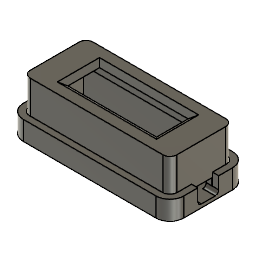
Slot na displej (Autodesk Fusion 360 design; units mm, degrees)
Autodesk Fusion 360 part; units mm, degrees
sketch "Sketch1" plane through (0, 0, 0) normal (0, 0, 1) x (1, 0, 0)
  line L0 (19.5, 10.25) -> (-18.5, 10.25)
  line L1 (-20.5, 8.25) -> (-20.5, -5.75)
  line L2 (-18.5, -7.75) -> (19.5, -7.75)
  line L3 (21.5, -5.75) -> (21.5, 8.25)
  line L4 (21.5, 10.25) -> (-20.5, -7.75) construction
  line L5 (-20.5, 10.25) -> (21.5, -7.75) construction
  line L6 (19.2, 6.275) -> (-19.2, 6.275)
  line L7 (-19.2, 6.275) -> (-19.2, -6.275)
  line L8 (-19.2, -6.275) -> (19.2, -6.275)
  line L9 (19.2, 6.275) -> (-19.2, -6.275) construction
  line L10 (-19.2, 6.275) -> (19.2, -6.275) construction
  arc A0 (21.5, 8.25) -> (19.5, 10.25) centre (19.5, 8.25) ccw
  arc A1 (19.5, -7.75) -> (21.5, -5.75) centre (19.5, -5.75) ccw
  arc A2 (-20.5, -5.75) -> (-18.5, -7.75) centre (-18.5, -5.75) ccw
  arc A3 (-18.5, 10.25) -> (-20.5, 8.25) centre (-18.5, 8.25) ccw
  line L11 (19.2, 2.9246) -> (13.2, 2.9246) construction
  line L12 (-19.2, 0) -> (-12.2, 0) construction
  line L13 (6.4271, 6.275) -> (6.4271, 5.775) construction
  line L14 (3.4944, -6.275) -> (3.4944, -3.275) construction
  line L15 (-12.2, -3.275) -> (13.2, -3.275)
  line L16 (13.2, -3.275) -> (13.2, 5.775)
  line L17 (13.2, 5.775) -> (-12.2, 5.775)
  line L18 (-12.2, 5.775) -> (-12.2, -3.275)
  line L19 (-13.7, -4.775) -> (14.7, -4.775)
  line L20 (14.7, -4.775) -> (14.7, 7.275)
  line L21 (14.7, 7.275) -> (-13.7, 7.275)
  line L22 (-13.7, 7.275) -> (-13.7, -4.775)
  line L23 (19.2, -6.275) -> (19.2, 2.725) construction
  line L24 (19.2, -6.275) -> (19.9, -6.275)
  line L25 (19.9, -6.275) -> (19.9, 2.725)
  line L26 (19.9, 2.725) -> (19.2, 2.725)
  line L27 (19.2, 6.275) -> (19.2, 2.725)
  line L28 (19.2, 6.275) -> (19.2, -6.275) construction
  line L29 (-12.2, -3.275) -> (13.2, 5.775) construction
  line L30 (-12.2, 5.775) -> (13.2, -3.275) construction
  point P0 (0.5, 1.25)
  point P1 (0.5, 1.25)
  dimension "d1" = 42
  dimension "d2" = 18
  dimension "d3" = 38.4
  dimension "d4" = 12.55
  dimension "d5" = 2
  dimension "d6" = 6
  dimension "d7" = 7
  dimension "d8" = 0.5
  dimension "d9" = 3
  dimension "d10" = 1.5
  dimension "d15" = 9
  dimension "d16" = 0.7
  constraint horizontal L0
  constraint perpendicular L0 L1
  constraint parallel L0 L2
  constraint parallel L1 L3
  constraint horizontal L6
  constraint perpendicular L6 L7
  constraint parallel L6 L8
  constraint coincident L9 origin
  constraint coincident L10 origin
  constraint coincident L4.start L0
  constraint coincident L4.start L3
  constraint tangent L0 A0
  constraint tangent L3 A0
  constraint coincident L5.end L3
  constraint coincident L5.end L2
  constraint tangent L3 A1
  constraint tangent L2 A1
  constraint equal A0 A1
  constraint coincident L4.end L2
  constraint coincident L4.end L1
  constraint tangent L2 A2
  constraint tangent L1 A2
  constraint equal A0 A2
  constraint coincident L5.start L1
  constraint coincident L5.start L0
  constraint tangent L1 A3
  constraint tangent L0 A3
  constraint equal A0 A3
  constraint midpoint L7 L12.start
  constraint perpendicular L7 L12
  constraint coincident L6 L13.start
  constraint perpendicular L6 L13
  constraint coincident L8 L14.start
  constraint perpendicular L8 L14
  constraint horizontal L15
  constraint vertical L16
  constraint horizontal L17
  constraint vertical L18
  constraint coincident L13.end L17
  constraint coincident L11.end L16
  constraint coincident L14.end L15
  constraint coincident L12.end L18
  constraint perpendicular L8 L23
  constraint perpendicular L24 L25
  constraint perpendicular L26 L27
  constraint perpendicular L8 L28
  constraint coincident L11.start L28
  constraint perpendicular L11 L16
  constraint perpendicular L25 L26
  constraint midpoint L29 P1
  constraint midpoint L4 P1
  constraint coincident P1 P0
  measures "d1" distance of L4.end L5.end
  measures "d2" distance of L5.start L4.end
  measures "d3" distance of L7.end L8.end
  measures "d4" distance of L6.end L7.end
  measures "d5" radius of A0
  measures "d6" distance of L11.start L11.end
  measures "d7" distance of L12.start L12.end
  measures "d8" distance of L13.start L13.end
  measures "d9" distance of L14.start L14.end
  measures "d15" distance of L8.end L23.end
  measures "d16" distance of L8.end L24.end
extrude "Extrude1" add sketch "Sketch1" against normal blind 1 contours L0 L1 L2 L3 A0 A1 A2 A3 | L6 L7 L8 L19 L20 L22 L24 L25 L26 L27 | L6 L19 L20 L22 | L6 L20 L21 L22 makes body 1
chamfer "Chamfer1" distance 1.5 distance2 1 4 edges at (-12.2, 1.25, 0) (0.5, 5.775, 0) (0.5, -3.275, 0) (13.2, 1.25, 0) measured on face at (-17.7333, 2.7583, 0) measured on face at (-17.7333, 2.7583, 0) measured on face at (-17.7333, 2.7583, 0) measured on face at (-17.7333, 2.7583, 0) on bodies 1
extrude "Extrude2" add sketch "Sketch1" along normal blind -3.2 and the other way blind 1 contours L0 L1 L2 L3 A0 A1 A2 A3 | L6 L20 L21 L22 bodies 1
sketch "Sketch2" plane through (0, 0, -3.2) normal (0, 0, -1) x (1, 0, 0)
  line L0 (-19.2, -6.275) -> (-19.2, 6.275)
  line L1 (-19.2, 6.275) -> (19.9, 6.275)
  line L2 (19.9, 6.275) -> (19.9, -2.725)
  line L3 (19.9, -2.725) -> (19.2, -2.725)
  line L4 (19.2, -2.725) -> (19.2, -6.275)
  line L5 (19.2, -6.275) -> (-19.2, -6.275)
  arc A0 (-20.5, -8.25) -> (-18.5, -10.25) centre (-18.5, -8.25) ccw
  line L6 (-18.5, -10.25) -> (19.5, -10.25)
  arc A1 (19.5, -10.25) -> (21.5, -8.25) centre (19.5, -8.25) ccw
  line L7 (21.5, -8.25) -> (21.5, 5.75)
  arc A2 (21.5, 5.75) -> (19.5, 7.75) centre (19.5, 5.75) ccw
  line L8 (19.5, 7.75) -> (-18.5, 7.75)
  arc A3 (-18.5, 7.75) -> (-20.5, 5.75) centre (-18.5, 5.75) ccw
  line L9 (-20.5, 5.75) -> (-20.5, -8.25)
  line L10 (-19.2, 6.275) -> (-19.2, -8.25)
  line L11 (-19.2, -8.25) -> (19.9, -8.25)
  line L12 (19.9, -8.25) -> (19.9, 6.275)
  line L13 (19.9, 6.275) -> (-19.2, 6.275)
  dimension "d22" = 1.6
  dimension "d23" = 1.3
  dimension "d24" = 2
  measures "d22" distance of L7 L12
  measures "d23" distance of L9 L10
  measures "d24" distance of L6 L11
extrude "Extrude3" add sketch "Sketch2" along normal blind 9.5 bodies 1
chamfer "Chamfer2" distance 2 distance2 2 1 edges at (0.35, 8.25, -3.2) measured on face at (6.6333, 7.5917, -3.2) on bodies 1
chamfer "Chamfer3" distance 0.7 distance2 2 1 edges at (19.9, 4.4875, -3.2) measured on face at (19.4333, 3.9, -3.2) on bodies 1
extrude "Extrude1'" add 1 faces at (-5.9333, 8.9167, -12.7) along direction (0, 0, -1) blind 2 separate body on bodies 1 makes body 2 in component "Component"
sketch "Sketch4" plane through (0, 0, -14.7) normal (0, 0, -1) x (1, 0, 0)
  line L0 (-19.2, 6.275) -> (19.9, 6.275)
  line L1 (19.9, 6.275) -> (19.9, -8.25)
  line L2 (19.9, -8.25) -> (-19.2, -8.25)
  line L3 (-19.2, -8.25) -> (-19.2, 6.275)
  line L4 (-20.5, 5.75) -> (-20.5, -8.25)
  arc A0 (-20.5, -8.25) -> (-18.5, -10.25) centre (-18.5, -8.25) ccw
  line L5 (-18.5, -10.25) -> (19.5, -10.25)
  arc A1 (19.5, -10.25) -> (21.5, -8.25) centre (19.5, -8.25) ccw
  line L6 (21.5, -8.25) -> (21.5, 5.75)
  arc A2 (21.5, 5.75) -> (19.5, 7.75) centre (19.5, 5.75) ccw
  line L7 (19.5, 7.75) -> (-18.5, 7.75)
  arc A3 (-18.5, 7.75) -> (-20.5, 5.75) centre (-18.5, 5.75) ccw
extrude "Extrude3'" add sketch "Sketch4" against normal blind 1 contours L0 L1 L2 L3 bodies 2 in component "Component"
sketch "Sketch5" plane through (21.5, 0, 0) normal (1, 0, 0) x (0, 1, 0)
  line L0 (8.25, -12.7) -> (-5.75, -12.7)
  line L1 (-5.75, -12.7) -> (-5.75, -14.7)
  line L2 (-5.75, -14.7) -> (8.25, -14.7)
  line L3 (8.25, -14.7) -> (8.25, -12.7)
  line L4 (8.25, -13.7) -> (-6.275, -13.7)
  line L5 (-6.275, -13.7) -> (8.25, -13.7)
  line L6 (1.25, -12.7) -> (-1.75, -12.6593) construction
  line L7 (-1.75, -10.7) -> (4.25, -10.7)
  line L8 (4.25, -10.7) -> (4.25, -12.7)
  line L9 (3.25, -13.7) -> (-0.75, -13.7)
  line L10 (-1.75, -12.7) -> (-1.75, -10.7)
  arc A0 (3.25, -13.7) -> (4.25, -12.7) centre (3.25, -12.7) ccw
  arc A1 (-1.75, -12.7) -> (-0.75, -13.7) centre (-0.75, -12.7) ccw
  line L11 (8.25, -12.7) -> (-5.75, -12.7) construction
  line L12 (1.25, -12.7) -> (1.25, -8.7) construction
  point P0 (-1.75, -13.7)
  dimension "d49" = 6
  dimension "d50" = 3
  dimension "d51" = 1
  constraint coincident L0.end L1.start
  constraint horizontal L7
  constraint vertical L8
  constraint horizontal L9
  constraint vertical L10
  constraint tangent L9 A0
  constraint tangent L8 A0
  constraint coincident P0 L9
  constraint coincident P0 L10
  constraint tangent L9 A1
  constraint tangent L10 A1
  constraint equal A0 A1
  constraint coincident L0.start L3.end
  constraint midpoint L6.start L11
  constraint coincident L8.start L7
  constraint coincident L8 L7.end
  constraint midpoint L7 L12
  constraint collinear L4 L9
  constraint perpendicular L11 L12
  measures "d49" distance of L7.start L7.end
  measures "d50" distance of L7.start P0
  measures "d51" radius of A0
extrude "Extrude4" cut sketch "Sketch5" against normal blind 2 contours L0 L4 L5 L9 A0 A1 | L0 L7 L8 L10 bodies 2 in component "Component"
copy_body "Body->Comp1" bodies 1 removing the originals makes body 3 in component "Component'"
extrude "Extrude1''" cut sketch "Sketch5" against normal blind 9 contours L0 L7 L8 L10 bodies 3 in component "Component'"
move_face "OffsetFaces1" offset 2 8 faces at (-5.8333, 10.25, -13.3667) (21.39, 8.9041, -14.0333) (6.8333, -7.75, -13.3667) (-20.5, -1.0833, -13.3667) (-18.9715, -7.6936, -14.0333) (-19.8802, 9.6975, -14.0333) (21.5, 6.9032, -13.4606) (19.9715, -7.6936, -14.0333) on bodies 2 in component "Component"
sketch "Sketch6" plane through (0, 0, -12.7) normal (0, 0, 1) x (-1, 0, 0)
  line L0 (-23.5, -4.25) -> (-23.5, -8.25)
  arc A0 (-23.5, -8.25) -> (-19.5, -12.25) centre (-19.5, -8.25) ccw
  line L1 (-19.5, -12.25) -> (18.5, -12.25)
  arc A1 (18.5, -12.25) -> (22.5, -8.25) centre (18.5, -8.25) ccw
  line L2 (22.5, -8.25) -> (22.5, 5.75)
  arc A2 (22.5, 5.75) -> (18.5, 9.75) centre (18.5, 5.75) ccw
  line L3 (18.5, 9.75) -> (-19.5, 9.75)
  arc A3 (-19.5, 9.75) -> (-23.5, 5.75) centre (-19.5, 5.75) ccw
  line L4 (-19.9, 1.75) -> (-19.9, 6.275)
  line L5 (-19.9, 6.275) -> (19.2, 6.275)
  line L6 (19.2, 6.275) -> (19.2, -8.25)
  line L7 (19.2, -8.25) -> (-19.9, -8.25)
  arc A4 (18.5, -10.25) -> (20.5, -8.25) centre (18.5, -8.25) ccw
  line L8 (20.5, -8.25) -> (20.5, 5.75)
  arc A5 (20.5, 5.75) -> (18.5, 7.75) centre (18.5, 5.75) ccw
  line L9 (18.5, 7.75) -> (-19.5, 7.75)
  arc A6 (-19.5, 7.75) -> (-21.5, 5.75) centre (-19.5, 5.75) ccw
  line L10 (-21.5, 5.75) -> (-21.5, -8.25)
  arc A7 (-21.5, -8.25) -> (-19.5, -10.25) centre (-19.5, -8.25) ccw
  line L11 (-19.5, -10.25) -> (18.5, -10.25)
  line L12 (13.7, 4.775) -> (13.7, -7.275)
  line L13 (13.7, -7.275) -> (-14.7, -7.275)
  line L14 (-14.7, -7.275) -> (-14.7, 4.775)
  line L15 (-14.7, 4.775) -> (13.7, 4.775)
  line L16 (-21.7, 5.75) -> (-21.7, -8.25)
  arc A8 (-21.7, -8.25) -> (-19.5, -10.45) centre (-19.5, -8.25) ccw
  line L17 (-19.5, -10.45) -> (18.5, -10.45)
  arc A9 (18.5, -10.45) -> (20.7, -8.25) centre (18.5, -8.25) ccw
  line L18 (20.7, -8.25) -> (20.7, 5.75)
  arc A10 (20.7, 5.75) -> (18.5, 7.95) centre (18.5, 5.75) ccw
  line L19 (18.5, 7.95) -> (-19.5, 7.95)
  arc A11 (-19.5, 7.95) -> (-21.7, 5.75) centre (-19.5, 5.75) ccw
  line L20 (-19.9, -4.25) -> (-23.5, -4.25)
  line L21 (-23.5, 5.75) -> (-23.5, 1.75)
  line L22 (-23.5, 1.75) -> (-19.9, 1.75)
  line L23 (-19.9, -8.25) -> (-19.9, -4.25)
  dimension "d57" = 0.2
extrude "Extrude5" add sketch "Sketch6" along normal blind 3.5 contours L0 A0 L1 A1 L2 A2 L3 A3 L16 A8 L17 A9 L18 A10 L19 A11 L20 L21 L22 bodies 2 in component "Component"
component "Component" placed x (1, 0, 0) y (0, 1, 0) z (0, 0, 1) at (0, 0, 0)
component "Component'" placed x (1, 0, 0) y (0, 1, 0) z (0, 0, 1) at (0, 0, 0)
equation "d25 = 14.7 mm - 3.2 mm - 5 mm + 2.5 mm + 0.5 mm"
